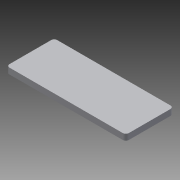
# Autodesk Inventor part: Support for bracket
Saved by Autodesk Inventor 2013 (Build 170138000, 138)
## iProperties
Created: 2013-01-31
Part Number: Support for bracket
Material: Aluminum 6061
Document SubType Name: Sheet Metal
Designer: aslane
Density: 1 g/cm^3
Sheet Metal Rule: Default
Author: aslane
Autodesk Inventor part; units mm, degrees
ref_plane "YZ Plane" through (0, 0, 0) normal (1, 0, 0) x (0, 1, 0)
ref_plane "XZ Plane" through (0, 0, 0) normal (0, 1, 0) x (-1, 0, 0)
ref_plane "XY Plane" through (0, 0, 0) normal (0, 0, 1) x (1, 0, 0)
sketch "Sketch1" plane through (0, 0, 0) normal (0, 1, 0) x (-1, 0, 0)
  arc A0 (-63.5, -23.8125) -> (-61.9125, -25.4) centre (-61.9125, -23.8125) ccw
  line L0 (-61.9125, -25.4) -> (-1.5875, -25.4)
  arc A1 (-1.5875, -25.4) -> (0, -23.8125) centre (-1.5875, -23.8125) ccw
  line L1 (0, -23.8125) -> (0, -1.5875)
  arc A2 (0, -1.5875) -> (-1.5875, 0) centre (-1.5875, -1.5875) ccw
  line L2 (-1.5875, 0) -> (-61.9125, 0)
  arc A3 (-61.9125, 0) -> (-63.5, -1.5875) centre (-61.9125, -1.5875) ccw
  line L3 (-63.5, -1.5875) -> (-63.5, -23.8125)
  circle A4 centre (-53.975, -12.7) radius 3.302
  circle A5 centre (-9.525, -12.7) radius 3.302
  point P0 (0, 0)
  point P1 (0, 0)
extrude "Plate1" add sketch "Sketch1" along normal blind 3.175 contours L3 A3 L2 A2 L1 A1 L0 A0 | A4 | A5
equation "\"BendRadius\" = Thickness"
equation "\"BendReliefWidth\" = Thickness"
equation "\"BendReliefDepth\" = 0.5 * Thickness"
equation "\"CornerReliefSize\" = 4 * Thickness"
equation "\"MinimumRemnant\" = 2 * Thickness"
equation "\"TransitionRadius\" = BendRadius"
equation "\"JacobiRadiusSize\" = BendRadius"
equation "\"GapSize\" = Thickness"
equation "\"d0\" = BendRadius"
equation "\"Thickness\" = 3.175"
body "Solid1"
